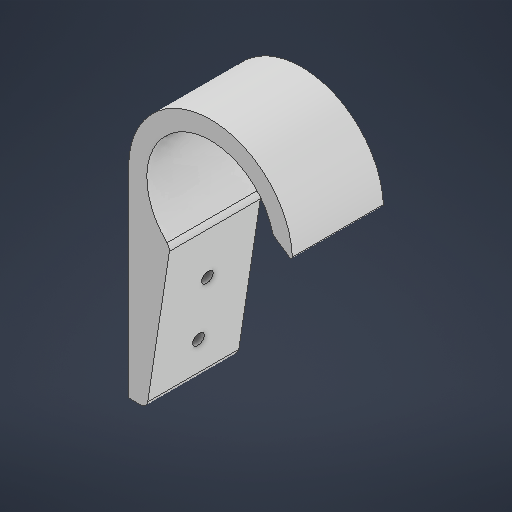
# Autodesk Inventor part: крюк старый
Saved by Autodesk Inventor 2025 (Build 290162000, 162)
## iProperties
Created: 2024-12-14
Part Number: крюк старый
Material: Типовые
Document SubType Name: Modeling
Designer: Phantom
Density: 1 g/cm^3
Appearance: По умолчанию
Author: Phantom
Autodesk Inventor part; units mm, degrees
ref_plane "YZ Plane" through (0, 0, 0) normal (1, 0, 0) x (0, 1, 0)
ref_plane "XZ Plane" through (0, 0, 0) normal (0, 1, 0) x (-1, 0, 0)
ref_plane "XY Plane" through (0, 0, 0) normal (0, 0, 1) x (1, 0, 0)
sketch "Эскиз1" plane through (0, 0, 0) normal (0, 0, 1) x (1, 0, 0)
  arc A0 (16.937, 4.4032) -> (-11.9308, -12.8026) centre (0, 0) ccw
  arc A1 (22.4785, 0.9844) -> (-22.5, 0) centre (0, 0) ccw
  line L0 (-22.5, 0) -> (-22.5, -55)
  line L1 (-22.5, 0) -> (32.5, 0) construction
  line L2 (-22.5, -55) -> (-17.5, -55)
  line L3 (21.6965, 0.5499) -> (17.743, 3.256)
  arc A2 (-11.3173, -14.5681) -> (-11.9308, -12.8026) centre (-13.2943, -14.2658) ccw
  arc A3 (16.937, 4.4032) -> (17.743, 3.256) centre (18.8727, 4.9064) ccw
  arc A4 (21.6965, 0.5499) -> (22.4785, 0.9844) centre (21.9789, 0.9626) ccw
  line L4 (-11.3173, -14.5681) -> (-17.5, -55)
  point P0 (22.5, 0)
  point P1 (-11.1519, -13.4865)
  point P2 (17.1061, 3.6919)
  dimension "d0" = 35
  dimension "d1" = 45
  dimension "d2" = 55
  dimension "d3" = 90
  dimension "d4" = 5
  dimension "d5" = 2
  dimension "d6" = 0.5
  constraints: 13 point on circle, 10 end point, 5 centre point, 5 tangent, 3 point on line, 2 coincident, 2 perpendicular, 1 equal radius, 1 horizontal, 1 vertical
  measures "d0" diameter of A0
  measures "d1" diameter of A1
  measures "d2" distance of L0.start L0.end
  measures "d3" angle of L0 L1
  measures "d4" distance of L0.end L2.end
  measures "d5" radius of A2
  measures "d6" radius of A4
extrude "Выдавливание1" add sketch "Эскиз1" along normal blind 25
fillet "Сопряжение3" radius 2 1 edges at (-17.5, -55, 12.5)
sketch "Эскиз6" plane through (-22.5, -55, 0) normal (-1, 0, 0) x (0, 0, 1)
  line L0 (25, 0) -> (0, 0) projected
  line L1 (12.5, 0) -> (12.5, 55)
  line L2 (0, 55) -> (25, 55) projected
  line L3 (0, 11) -> (25, 11)
  line L4 (0, 27) -> (25, 27)
  circle A0 centre (12.5, 27) radius 1.6
  circle A1 centre (12.5, 11) radius 1.6
  dimension "d30" = 11
  dimension "d32" = 16
  dimension "d33" = 3.2
  dimension "d34" = 3.2
  constraints: 6 end point, 4 midpoint, 2 centre point, 1 perpendicular
  measures "d30" distance between parallel lines of L0 L3
  measures "d32" distance between parallel lines of L3 L4
  measures "d33" diameter of A0
  measures "d34" diameter of A1
extrude "Выдавливание6" cut sketch "Эскиз6" against normal through all
